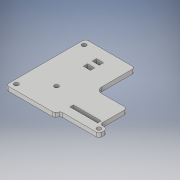
# Autodesk Inventor part: coxa
Saved by Autodesk Inventor 2019 (Build 230136000, 136)
## iProperties
Created: 2023-04-15
Part Number: coxa
Material: Generic
Document SubType Name: Modeling
Designer: Analuam
Density: 1 g/cm^3
Appearance: Default
Author: Analuam
Autodesk Inventor part; units mm, degrees
ref_plane "YZ Plane" through (0, 0, 0) normal (1, 0, 0) x (0, 1, 0)
ref_plane "XZ Plane" through (0, 0, 0) normal (0, 1, 0) x (-1, 0, 0)
ref_plane "XY Plane" through (0, 0, 0) normal (0, 0, 1) x (1, 0, 0)
sketch "Sketch1" plane through (0, 0, 0) normal (0, 1, 0) x (-1, 0, 0)
  line L0 (19.2289, 19.6338) -> (19.2289, -32.3662)
  line L1 (17.2289, -34.3662) -> (-13.7711, -34.3662)
  line L2 (-15.7711, -32.3662) -> (-15.7711, -10.826)
  line L3 (-19.7711, -6.826) -> (-35.887, -6.826)
  line L4 (-37.887, -4.826) -> (-37.887, 10.574)
  line L5 (17.2289, 21.6338) -> (-13.3861, 21.6338)
  line L6 (-14.943, 20.8893) -> (-16.2097, 19.3185)
  line L7 (-17.7665, 18.574) -> (-35.887, 18.574)
  line L8 (-16.8101, 12.574) -> (-36.4101, 12.574)
  line L9 (-36.4101, 12.574) -> (-36.4101, 10.174)
  line L10 (-36.4101, 10.174) -> (-16.8101, 10.174)
  line L11 (-16.8101, 10.174) -> (-16.8101, 12.574)
  arc A0 (19.2289, 19.6338) -> (17.2289, 21.6338) centre (17.2289, 19.6338) ccw
  arc A1 (17.2289, -34.3662) -> (19.2289, -32.3662) centre (17.2289, -32.3662) ccw
  arc A2 (-15.7711, -32.3662) -> (-13.7711, -34.3662) centre (-13.7711, -32.3662) ccw
  arc A3 (-15.7711, -10.826) -> (-19.7711, -6.826) centre (-19.7711, -10.826) ccw
  arc A4 (-37.887, -4.826) -> (-35.887, -6.826) centre (-35.887, -4.826) ccw
  arc A5 (-17.7665, 18.574) -> (-16.2097, 19.3185) centre (-17.7665, 20.574) ccw
  arc A6 (-13.3861, 21.6338) -> (-14.943, 20.8893) centre (-13.3861, 19.6338) ccw
  line L12 (-33.327, 18.574) -> (-41.327, 18.574)
  line L13 (-43.327, 16.574) -> (-43.327, 14.574)
  line L14 (-41.327, 12.574) -> (-39.887, 12.574)
  circle A7 centre (-40.327, 15.574) radius 1.5
  arc A8 (-37.887, 10.574) -> (-39.887, 12.574) centre (-39.887, 10.574) ccw
  arc A9 (-43.327, 14.574) -> (-41.327, 12.574) centre (-41.327, 14.574) ccw
  arc A10 (-41.327, 18.574) -> (-43.327, 16.574) centre (-41.327, 16.574) ccw
  circle A11 centre (16.0065, 17.5338) radius 1.5
  circle A12 centre (16.0065, -30.2662) radius 1.5
  circle A13 centre (0.5532, 4.6338) radius 1.5
  line L15 (3.2844, -26.2176) -> (-1.7156, -26.2176)
  line L16 (-1.7156, -26.2176) -> (-1.7156, -23.2176)
  line L17 (-1.7156, -23.2176) -> (3.2844, -23.2176)
  line L18 (3.2844, -23.2176) -> (3.2844, -26.2176)
  line L19 (3.2844, -20.0075) -> (-1.7156, -20.0075)
  line L20 (-1.7156, -20.0075) -> (-1.7156, -17.0075)
  line L21 (-1.7156, -17.0075) -> (3.2844, -17.0075)
  line L22 (3.2844, -17.0075) -> (3.2844, -20.0075)
  point P0 (0, 0)
  point P1 (-43.327, 12.574)
  dimension "d5" = 19.6
  dimension "d6" = 2.4
  dimension "d7" = 17
  dimension "d8" = 6
  dimension "d9" = 56
  dimension "d11" = 2
  dimension "d12" = 4
  dimension "d14" = 3
  dimension "d15" = 2
  dimension "d16" = 3
  dimension "d17" = 35
  dimension "d18" = 3
  dimension "d19" = 3
  dimension "d23" = 5
  dimension "d24" = 3
  dimension "d25" = 5
  dimension "d26" = 3
  constraints: 46 end point, 20 point on circle, 20 tangent, 14 centre point, 9 perpendicular, 7 equal radius, 7 parallel, 5 horizontal, 3 point on line, 1 vertical
  measures "d5" distance of L10.end L9.end
  measures "d6" distance of L9.end L8.end
  measures "d7" distance between parallel lines of L3 L10
  measures "d8" distance between parallel lines of L7 L8
  measures "d9" distance between parallel lines of L1 L5
  measures "d11" radius of A0
  measures "d12" radius of A3
  measures "d14" diameter of A7
  measures "d15" radius of A8
  measures "d16" distance from line of L13 A7.centre
  measures "d17" distance between parallel lines of L0 L2
  measures "d18" diameter of A11
  measures "d19" diameter of A13
  measures "d23" distance of L16.end L17.end
  measures "d24" distance of L15.end L16.end
  measures "d25" distance of L21.start L22.start
  measures "d26" distance of L19.end L21.start
sketch "Sketch2" plane through (0, 0, 0) normal (0, 1, 0) x (-1, 0, 0)
  point P0 (0, 0)
extrude "Extrusion2" add sketch "Sketch1" along normal blind 3
body "Solid2"
